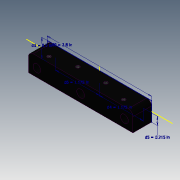
# Autodesk Inventor part: J005362
Saved by Autodesk Inventor 2015 SP1 (Build 190203100, 203)
## iProperties
Created: 2015-08-04
Material: ALUMINUM, 6061-T651
Vendor: HHMI: JRC - ID&F
Document SubType Name: Modeling
Designer: ARNOLDJ
Density: 2.7 g/cm^3
Appearance: Anodized - Black
Mass: 11.5747 g
Surface Area: 48.3947 cm^2
Volume: 9.8929 cm^3
Part Number: J005362
Description: MOUNT STEEL LOCK PLATE TO POSITIONER
Project: P-201804
RuleStatus: InUse
AfterDocSave0: file://Part Number Cleaner
LAB/DEPT: SVOBODA (LAB)
REQUESTING SCIENTIST: SOFRONIEW, NICK
SURFACE ROUGHNESS: 63 Ra
DESIGN DEPARTMENT: HHMI: JRC - ID&F
SPECIAL FINISH: ANODIZE PER MIL-A-8625F, TYPE II, CLASS 2 (BLACK)
ALTERED ITEM PART NUMBER: N/A
ALTERED ITEM VENDOR: N/A
ALTERED ITEM DESCRIPTION: N/A
Revision Number: -
Autodesk Inventor part; units mm, degrees
ref_plane "YZ Plane" through (0, 0, 0) normal (1, 0, 0) x (0, 1, 0)
ref_plane "XZ Plane" through (0, 0, 0) normal (0, 1, 0) x (-1, 0, 0)
ref_plane "XY Plane" through (0, 0, 0) normal (0, 0, 1) x (1, 0, 0)
sketch "Sketch1" plane through (0, 0, 0) normal (0, 0, 1) x (1, 0, 0)
  line L0 (35.56, -6.35) -> (-35.56, -6.35)
  line L1 (-35.56, -6.35) -> (-35.56, 6.35)
  line L2 (-35.56, 6.35) -> (35.56, 6.35)
  line L3 (35.56, 6.35) -> (35.56, -6.35)
  line L4 (35.56, -6.35) -> (-35.56, 6.35) construction
  line L5 (-35.56, -6.35) -> (35.56, 6.35) construction
  line L6 (0, 8.89) -> (0, -8.89) projected
  line L7 (-49.784, 0) -> (49.784, 0) projected
  point P0 (0, 0)
  point P1 (-29.845, -0.889)
  point P2 (0, -0.889)
  point P3 (29.845, -0.889)
  point P4 (0, 0)
  dimension "d0" = 71.12
  dimension "d1" = 12.7
  dimension "d4" = 29.845
  dimension "d5" = 5.461
  dimension "d6" = 29.845
  constraints: 12 end point, 3 midpoint, 2 horizontal alignment, 2 parallel, 1 horizontal, 1 perpendicular, 1 vertical alignment
  measures "d0" distance of L1.end L2.end
  measures "d1" distance of L0.end L1.end
  measures "d4" distance of point (0, -0.889) point (29.845, -0.889)
  measures "d5" distance from line of point (29.845, -0.889) L0
  measures "d6" distance of point (0, -0.889) point (-29.845, -0.889)
extrude "Extrusion1" add sketch "Sketch1" along normal blind 12.7
hole "Hole1" at (-29.845, -0.889, 0) at (0, -0.889, 0) at (29.845, -0.889, 0) direction (0, 0, 1) diameter 5.2578 end through all counterbore diameter 9.525 counterbore depth 5.08
sketch "Sketch2" plane through (0, 0, 0) normal (1, 0, 0) x (0, 1, 0)
  line L0 (-6.35, 0) -> (-6.35, 12.7) projected
  line L1 (-6.35, 12.7) -> (6.35, 12.7) projected
  line L2 (-6.35, 12.7) -> (-7.112, 12.7)
  line L3 (-7.112, 12.7) -> (-7.112, 13.462)
  line L4 (-7.112, 13.462) -> (-6.35, 13.462)
  line L5 (-6.35, 13.462) -> (-6.35, 15.24)
  line L6 (-6.35, 15.24) -> (-8.89, 15.24)
  line L7 (-8.89, 15.24) -> (-8.89, 10.795)
  line L8 (-8.89, 10.795) -> (-6.35, 8.255)
  line L9 (-6.35, 8.255) -> (-6.35, 12.7)
  point P0 (0, 0)
  dimension "d15" = 0.762
  dimension "d16" = 0.762
  dimension "d17" = 2.54
  dimension "d18" = 2.54
  dimension "d19" = 45
  dimension "d20" = 4.445
  constraints: 16 end point, 6 perpendicular, 2 point on line, 1 vertical alignment
  measures "d15" distance of L0.end L2.end
  measures "d16" distance of L2.end L3.end
  measures "d17" distance of L5.end L6.end
  measures "d18" distance between parallel lines of L1 L6
  measures "d19" angle of L0 L8
  measures "d20" distance from line of L8.end L1
extrude "Extrusion2" [suppressed]
sketch "Sketch3" plane through (-35.56, -6.35, 0) normal (0, -1, 0) x (1, 0, 0)
  line L0 (35.56, 15.24) -> (35.56, -2.54) projected
  line L1 (-14.224, 0) -> (85.344, 0) projected
  point P0 (35.56, 0)
  point P1 (26.035, 5.08)
  point P2 (45.085, 5.08)
  point P3 (10.16, 8.89)
  point P4 (60.96, 8.89)
  dimension "d23" = 9.525
  dimension "d24" = 9.525
  dimension "d35" = 8.89
  dimension "d36" = 8.89
  dimension "d37" = 5.08
  dimension "d38" = 15.875
  dimension "d39" = 15.875
  constraints: 1 horizontal alignment
  measures "d23" distance from line of L0 point (26.035, 5.08)
  measures "d24" distance from line of L0 point (45.085, 5.08)
  measures "d35" distance from line of point (10.16, 8.89) L1
  measures "d36" distance from line of point (60.96, 8.89) L1
  measures "d37" distance from line of L1 point (26.035, 5.08)
  measures "d38" horizontal distance of point (26.035, 5.08) point (10.16, 8.89)
  measures "d39" horizontal distance of point (45.085, 5.08) point (60.96, 8.89)
hole "Hole2" at (25.4, -6.35, 8.89) at (9.525, -6.35, 5.08) at (-9.525, -6.35, 5.08) at (-25.4, -6.35, 8.89) direction (0, 1, 0) diameter 2.4638 end through all
fillet "Fillet1" radius 3.175 2 edges at (35.56, 6.35, 6.35) (-35.56, 6.35, 6.35)
body "Solid1"
